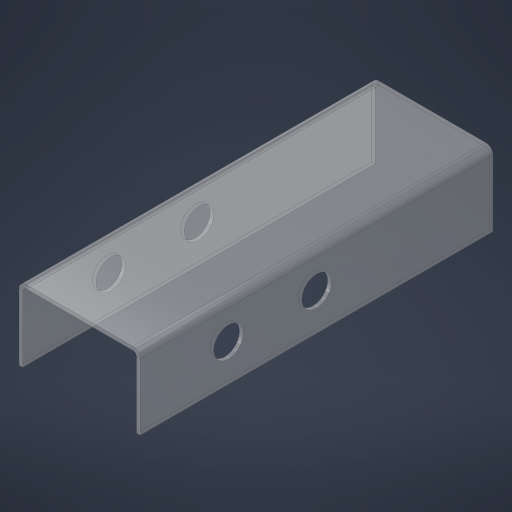
# Autodesk Inventor part: GP3-001
Saved by Autodesk Inventor 2023.4 (Build 274418000, 418)
## iProperties
Created: 2025-01-14
Part Number: GP3-001
Material: Polycarbonate, Clear
Document SubType Name: Sheet Metal
Designer: brand
Density: 1.2 g/cm^3
Sheet Metal Rule: Default
Appearance: Polycarbonate - Clear
Author: brand
Autodesk Inventor part; units mm, degrees
ref_plane "YZ Plane" through (0, 0, 0) normal (1, 0, 0) x (0, 1, 0)
ref_plane "XZ Plane" through (0, 0, 0) normal (0, 1, 0) x (-1, 0, 0)
ref_plane "XY Plane" through (0, 0, 0) normal (0, 0, 1) x (1, 0, 0)
sketch "Sketch1" plane through (0, 0, 0) normal (0, 1, 0) x (-1, 0, 0)
  line L0 (52.3875, -152.4) -> (-52.3875, -152.4)
  line L1 (-52.3875, -152.4) -> (-52.3875, 152.4)
  line L2 (-52.3875, 152.4) -> (52.3875, 152.4)
  line L3 (52.3875, 152.4) -> (52.3875, -152.4)
  line L4 (52.3875, -152.4) -> (-52.3875, 152.4) construction
  line L5 (-52.3875, -152.4) -> (52.3875, 152.4) construction
  point P0 (0, 0)
  dimension "d0" = 304.8
  dimension "d1" = 104.775
  measures "d0" distance of L2.end L0.start
  measures "d1" distance of L1.end L2.end
extrude "Plate1" add sketch "Sketch1" along normal mid plane 3.175
sketch "Sketch3" plane through (49.2125, 1.5875, 152.4) normal (1, 0, 0) x (0, 1, 0)
  line L0 (0, -304.8) -> (0, 0)
  line L1 (0, 0) -> (-63.5, 0)
  line L2 (-63.5, 0) -> (-63.5, -304.8)
  line L3 (-63.5, -304.8) -> (0, -304.8)
  constraints: 6 end point, 1 horizontal, 1 perpendicular, 1 vertical
edge flange "Flange1" height 63.5 angle 90 thickness 3.175 bend radius 3.175 thickness toward (1, 0, 0) relief straight relief width 3.175 relief depth 1.5875 corner gap 3.175 corner form 0 edges at (52.3875, -1.5875, 0) (-52.3875, -1.5875, 0) wall of the first edge with corners at (49.2125, 1.5875, -152.4) (49.2125, 1.5875, 152.4) (49.2125, -61.9125, 152.4) (49.2125, -61.9125, -152.4)
bend "Bend1"
corner "Corner1"
sketch "Sketch4" plane through (52.3875, -61.9125, 152.4) normal (1, 0, 0) x (0, 0, -1)
  line L0 (0, 63.5) -> (304.8, 63.5) construction
  line L1 (0, 0) -> (0, 57.15) construction
  point P0 (152.4, 61.9125)
  point P1 (76.2, 31.75)
  point P2 (152.4, 31.75)
  dimension "d14" = 31.75
  dimension "d15" = 76.2
  dimension "d16" = 76.2
  constraints: 1 horizontal alignment
  measures "d14" distance from line of point (76.2, 31.75) L0
  measures "d15" distance of point (152.4, 31.75) point (76.2, 31.75)
  measures "d16" distance from line of L1 point (76.2, 31.75)
hole "Hole1" at (52.3875, -30.1625, 76.2) at (52.3875, -30.1625, 0) direction (-1, 0, 0) diameter 25.4 end through all
equation "\"d22\" = Thickness"
equation "\"d2\" = Thickness"
equation "\"d4\" = BendReliefWidth"
equation "\"d5\" = BendReliefDepth"
equation "\"d6\" = MinimumRemnant"
equation "\"d7\" = TransitionRadius"
equation "\"d10\" = BendRadius"
equation "\"d11\" = CornerReliefSize"
equation "\"d12\" = GapSize"
equation "\"d13\" = JacobiRadiusSize"
equation "\"BendRadius\" = Thickness"
equation "\"BendReliefWidth\" = Thickness"
equation "\"BendReliefDepth\" = 0.5 * Thickness"
equation "\"CornerReliefSize\" = 4 * Thickness"
equation "\"MinimumRemnant\" = 2 * Thickness"
equation "\"TransitionRadius\" = BendRadius"
equation "\"JacobiRadiusSize\" = BendRadius"
equation "\"GapSize\" = Thickness"
equation "\"Thickness\" = 3.175"
body "Solid1"
